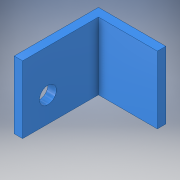
# Autodesk Inventor part: Cylinder mount
Saved by Autodesk Inventor 2017 (Build 210142000, 142)
## iProperties
Created: 2017-01-19
Part Number: Cylinder mount
Material: Generic
Document SubType Name: Modeling
Designer: Ben
Density: 1 g/cm^3
Appearance: Cyan
Author: Ben
Autodesk Inventor part; units mm, degrees
ref_plane "YZ Plane" through (0, 0, 0) normal (1, 0, 0) x (0, 1, 0)
ref_plane "XZ Plane" through (0, 0, 0) normal (0, 1, 0) x (-1, 0, 0)
ref_plane "XY Plane" through (0, 0, 0) normal (0, 0, 1) x (1, 0, 0)
sketch "Sketch1" plane through (0, 0, 0) normal (0, 1, 0) x (-1, 0, 0)
  line L0 (0, 31.75) -> (0, 0)
  line L1 (0, 0) -> (-25.4, 0)
  line L2 (-25.4, 0) -> (-25.4, 3.175)
  line L3 (-25.4, 3.175) -> (-3.175, 3.175)
  line L4 (-3.175, 3.175) -> (-3.175, 31.75)
  line L5 (-3.175, 31.75) -> (0, 31.75)
  dimension "d0" = 31.75
  dimension "d1" = 25.4
  dimension "d2" = 3.175
  constraints: 12 end point, 6 perpendicular, 1 vertical
  measures "d0" distance of L0.start L0.end
  measures "d1" distance of L0.end L1.end
  measures "d2" distance of L4.end L0.start
extrude "Extrusion1" add sketch "Sketch1" along normal blind 25.4
sketch "Sketch2" plane through (3.175, 0, 31.75) normal (1, 0, 0) x (0, 0, -1)
  circle A0 centre (9.525, 9.525) radius 3.175
  line L0 (31.75, 0) -> (31.75, 25.4) construction
  line L1 (0, 0) -> (28.575, 0) construction
  dimension "d5" = 6.35
  dimension "d6" = 22.225
  dimension "d7" = 9.525
  constraints: 1 centre point
  measures "d5" diameter of A0
  measures "d6" distance from line of L0 A0.centre
  measures "d7" distance from line of L1 A0.centre
extrude "Extrusion2" cut sketch "Sketch2" against normal through all
body "Solid1"
